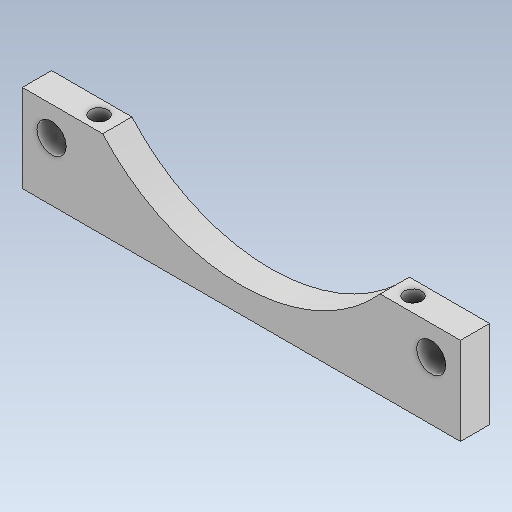
# Autodesk Inventor part: Tank Holder
Saved by Autodesk Inventor 2021 (Build 250183000, 183)
## iProperties
Created: 2022-01-12
Part Number: Tank Holder
Material: Generic
Document SubType Name: Modeling
Designer: Alex Clay
Density: 1 g/cm^3
Appearance: Default
Author: Alex Clay
Autodesk Inventor part; units mm, degrees
ref_plane "YZ Plane" through (0, 0, 0) normal (1, 0, 0) x (0, 1, 0)
ref_plane "XZ Plane" through (0, 0, 0) normal (0, 1, 0) x (-1, 0, 0)
ref_plane "XY Plane" through (0, 0, 0) normal (0, 0, 1) x (1, 0, 0)
sketch "Sketch1" plane through (0, 0, 0) normal (0, 0, 1) x (1, 0, 0)
  line L0 (-190.5, 76.2) -> (-190.5, 0)
  line L1 (-190.5, 0) -> (190.5, 0)
  line L2 (190.5, 0) -> (190.5, 76.2)
  line L3 (190.5, 76.2) -> (120.6918, 76.2)
  line L4 (-190.5, 76.2) -> (-120.6918, 76.2)
  arc A0 (-120.6918, 76.2) -> (120.6918, 76.2) centre (0, 184.15) ccw
  point P0 (0, 0)
  point P1 (0, 0)
  dimension "d0" = 161.925
  dimension "d1" = 381
  dimension "d2" = 190.5
  dimension "d3" = 76.2
  dimension "d4" = 184.15
  constraints: 10 end point, 2 horizontal, 2 midpoint, 2 point on circle, 2 vertical, 1 centre point, 1 collinear, 1 parallel, 1 vertical alignment
  measures "d0" radius of A0
  measures "d1" distance of L0.end L1.end
  measures "d2" distance from line of point (0, 0) L0
  measures "d3" distance of L1.end L2.end
  measures "d4" distance from line of L1 A0.centre
extrude "Extrusion1" add sketch "Sketch1" along normal mid plane 25.4
sketch "Sketch2" plane through (-190.5, 76.2, 12.7) normal (0, 1, 0) x (1, 0, 0)
  line L0 (0, 25.4) -> (69.8082, 0) construction
  line L1 (69.8082, 0) -> (0, 0) projected
  line L2 (69.8082, 25.4) -> (69.8082, 0) projected
  line L3 (0, 0) -> (0, 25.4) projected
  line L4 (0, 25.4) -> (69.8082, 25.4) projected
  line L5 (0, 0) -> (69.8082, 25.4) construction
  point P0 (53.9541, 12.7)
  point P1 (34.9041, 12.7)
  dimension "d14" = 19.05
  constraints: 8 point on line, 4 end point, 1 horizontal alignment, 1 midpoint
  measures "d14" distance of point (53.954, 12.7) point (34.904, 12.7)
hole "Hole1" at (-136.5459, 76.2, 0) direction (0, -1, 0) diameter 8.89 end through all counterbore diameter 15.24 counterbore depth 27.94 clearance for "Socket Head Cap Screw" size "M8" standard "Ansi Metric M Profile"
sketch "Sketch3" plane through (0, 0, 12.7) normal (0, 0, 1) x (1, 0, 0)
  line L0 (-120.6918, 76.2) -> (-190.5, 76.2) projected
  line L1 (-190.5, 76.2) -> (-190.5, 0) projected
  point P0 (0, 0)
  point P1 (-165.1, 50.8)
  dimension "d23" = 25.4
  dimension "d24" = 25.4
  measures "d23" distance from line of point (-165.1, 50.8) L0
  measures "d24" distance from line of point (-165.1, 50.8) L1
hole "Hole2" at (-165.1, 50.8, 12.7) direction (0, 0, -1) diameter 25.4 end through all
mirror "Mirror1" about plane through (0, 0, 0) normal (1, 0, 0) of "Hole1", "Hole2"
equation "\"d2\" = 0.5 * d1"
body "Solid1"
